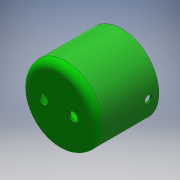
# Autodesk Inventor part: cuerpo
Saved by Autodesk Inventor 2016 (Build 200138000, 138)
## iProperties
Created: 2016-02-19
Part Number: cuerpo
Material: Genérico
Document SubType Name: Modeling
Designer: Usuario1
Density: 1 g/cm^3
Appearance: Valor por defecto
Author: Usuario1
Autodesk Inventor part; units mm, degrees
ref_plane "XZ Plane" through (0, 0, 0) normal (0, 1, 0) x (-1, 0, 0)
ref_plane "XY Plane" through (0, 0, 0) normal (0, 0, 1) x (1, 0, 0)
sketch "Boceto1" plane through (0, 0, 0) normal (0, 0, 1) x (1, 0, 0)
  line L0 (0, 0) -> (-4.6715, 0)
  line L1 (-5.8393, 9.9269) -> (-5.8393, 1.1679)
  line L2 (-5.5393, 9.6269) -> (-5.5393, 1.1679)
  arc A0 (-5.8393, 1.1679) -> (-4.6715, 0) centre (-4.6715, 1.1679) ccw
  arc A1 (-5.5393, 1.1679) -> (-4.6715, 0.3) centre (-4.6715, 1.1679) ccw
  line L3 (0, 0) -> (-4.6715, 0)
  line L4 (0, 0.3) -> (-4.6715, 0.3)
  line L5 (0, 0.3) -> (0, 0)
  line L6 (-5.8393, 9.9269) -> (-5.5393, 9.6269)
  constraints: 14 end point, 4 point on circle, 2 centre point
revolve "Revolución1" add sketch "Boceto1" angle 360 about axis through (0, 0.3, 0) along (0, -1, 0)
sketch "Boceto2" plane through (0, 0, 0) normal (1, 0, 0) x (0, 1, 0)
  line L0 (9.6269, 5.5393) -> (1.1679, 5.5393) projected
  line L1 (9.6269, -5.5393) -> (1.1679, -5.5393) projected
  line L2 (9.6269, 5.5393) -> (9.6269, 4.0393)
  line L3 (9.6269, -5.5393) -> (9.6269, 5.5393) projected
  line L4 (9.6269, 4.0393) -> (7.1269, 4.0393)
  line L5 (7.1269, 4.0393) -> (7.1269, 5.5393)
  line L6 (9.6269, 5.5393) -> (7.1269, 5.5393)
  line L7 (9.6269, 0) -> (13.8106, 0)
  line L8 (9.6269, -5.5393) -> (9.6269, -4.0393)
  line L9 (9.6269, -4.0393) -> (7.1269, -4.0393)
  line L10 (7.1269, -4.0393) -> (7.1269, -5.5393)
  point P0 (0, 0)
  dimension "d1" = 1.5
  dimension "d2" = 2.5
  dimension "d3" = 1.5
  dimension "d4" = 2.5
  constraints: 16 end point, 5 perpendicular, 4 point on line, 1 horizontal, 1 midpoint
  measures "d1" distance of L0.start L2.end
  measures "d2" distance of L2.end L4.end
  measures "d3" distance of L1.start L8.end
  measures "d4" distance of L8.end L9.end
revolve "Revolución2" add sketch "Boceto2" angle 30 mid plane about axis through (0, 9.6269, 0) along (0, 1, 0)
sketch "Boceto3" plane through (0, 9.6269, 0) normal (0, 1, 0) x (1, 0, 0)
  line L0 (-1.0455, -3.9017) -> (-1.4337, -5.3506) projected
  arc A0 (-1.4337, -5.3506) -> (1.4337, -5.3506) centre (0, 0) ccw projected
  line L1 (1.0455, -3.9017) -> (1.4337, -5.3506) projected
  arc A1 (-1.0455, -3.9017) -> (1.0455, -3.9017) centre (0, 0) ccw projected
  line L2 (1.4337, 5.3506) -> (1.0455, 3.9017) projected
  arc A2 (1.4337, 5.3506) -> (-1.4337, 5.3506) centre (0, 0) ccw projected
  line L3 (-1.0455, 3.9017) -> (-1.4337, 5.3506) projected
  arc A3 (1.0455, 3.9017) -> (-1.0455, 3.9017) centre (0, 0) ccw projected
  circle A4 centre (0, 4.7895) radius 0.6
  circle A5 centre (0, -4.7895) radius 0.6
  dimension "d9" = 1.2
  dimension "d10" = 1.2
  constraints: 2 centre point
  measures "d9" diameter of A4
  measures "d10" diameter of A5
extrude "Extrusión1" add sketch "Boceto3" along normal blind 0.155 contours A4 | A5
ref_plane "Plano de trabajo1" through (-8, 0, 0) normal (1, 0, 0) x (0, 1, 0)
sketch "Boceto6" plane through (-8, 0, 0) normal (1, 0, 0) x (0, 1, 0)
  line L0 (1.1679, -5.8393) -> (1.1679, 5.8393) projected
  line L1 (9.9269, -5.8393) -> (9.9269, 5.8393) projected
  line L2 (0, -4.6715) -> (0, 4.6715) projected
  line L3 (1.1679, -5.8393) -> (1.1679, 5.8393) projected
  circle A0 centre (8.2551, 0) radius 0.55
  point P0 (0, 0)
  constraints: 1 centre point
extrude "Extrusión2" cut sketch "Boceto6" along normal blind 16
sketch "Boceto7" plane through (0, 0, 0) normal (0, -1, 0) x (1, 0, 0)
  circle A0 centre (-2.3358, 0) radius 0.7
  circle A1 centre (2.3358, 0) radius 0.7
  point P0 (0, 0)
  dimension "d17" = 1.4
  dimension "d18" = 1.4
  constraints: 2 centre point
  measures "d17" diameter of A0
  measures "d18" diameter of A1
extrude "Extrusión3" cut sketch "Boceto7" against normal blind 3
